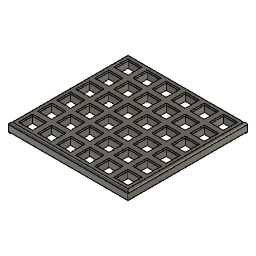
Parametric_Key_Tester (Autodesk Fusion 360 design; units mm, degrees)
part number: Parametric Key Tester
Autodesk Fusion 360 part; units mm, degrees
sketch "Sketch1" plane through (0, 0, 0) normal (0, 0, 1) x (1, 0, 0) in component "Key Tester"
  line L0 (0, 0) -> (119, 0)
  line L1 (119, 0) -> (119, 119)
  line L2 (119, 119) -> (0, 119)
  line L3 (0, 119) -> (0, 0)
  line L4 (5, 5) -> (19, 5)
  line L5 (19, 5) -> (19, 19)
  line L6 (19, 19) -> (5, 19)
  line L7 (5, 19) -> (5, 5)
  line L8 (4, 4) -> (20, 4)
  line L9 (20, 4) -> (20, 20)
  line L10 (20, 20) -> (4, 20)
  line L11 (4, 20) -> (4, 4)
  dimension "d1" = 119
  dimension "d2" = 119
  dimension "d3" = 14
  dimension "d4" = 14
  dimension "d5" = 5
  dimension "d6" = 5
  dimension "d65" = 1
  constraint horizontal L0
  constraint vertical L1
  constraint coincident L0.start L3.end
  constraint horizontal L4
  constraint vertical L5
  constraint horizontal L6
  constraint vertical L7
  constraint horizontal L2
  measures "d1" distance of L0.start L0.end
  measures "d2" distance of L0.start L2.end
  measures "d3" distance of L4.start L4.end
  measures "d4" distance of L4.start L6.end
  measures "d5" distance of L3 L7
  measures "d6" distance of L0 L4
extrude "Extrude6" add sketch "Sketch1" along normal blind 10 contours L0 L1 L2 L3 | L4 L5 L6 L7 | L8 L9 L10 L11 in component "Key Tester"
fillet "Fillet3" radius 2 8 edges at (59.5, 119, 10) (0, 59.5, 10) (59.5, 0, 10) (119, 59.5, 10) (59.5, 119, 0) (119, 59.5, 0) (0, 59.5, 0) (59.5, 0, 0) in component "Key Tester"
extrude "Extrude7" cut sketch "Sketch1" along normal up to surface (10 mm away) contours L4 L5 L6 L7 in component "Key Tester"
extrude "Extrude8" cut sketch "Sketch1" along normal up to surface (8.2 mm away) contours L8 L9 L10 L11 in component "Key Tester"
fillet "Fillet4" radius 1 4 edges at (12, 20, 0) (20, 12, 0) (12, 4, 0) (4, 12, 0) in component "Key Tester"
pattern_linear "R-Pattern1" count 6 spacing 19 along (0, 1, 0) count 6 spacing 19 along (1, 0, 0) of "Extrude7", "Extrude8", "Fillet4" in component "Key Tester"
component "Key Tester" placed x (1, 0, 0) y (0, 1, 0) z (0, 0, 1) at (0, 0, 0)
equation "d1 = SwitchWidth * Columns + SwitchSpacing * Columns + SwitchSpacing"
equation "d2 = SwitchHeight * Rows + SwitchSpacing * Rows + SwitchSpacing"
equation "d3 = SwitchWidth"
equation "d4 = SwitchHeight"
equation "d5 = SwitchSpacing"
equation "d6 = SwitchSpacing"
equation "Rows = 6" comment "Number of rows"
equation "Columns = 6" comment "Number of columns"
equation "SwitchHeight = 14 mm" comment "Switch Height (14 for MX)"
equation "SwitchWidth = 14 mm" comment "Switch Width (14 for MX)"
equation "SwitchSpacing = 5 mm" comment "Spacing between switches (Normally 5)"
equation "d68 = Thickness"
equation "d78 = Rows"
equation "d79 = Columns"
equation "d80 = -( SwitchWidth + SwitchSpacing )"
equation "d81 = -( SwitchWidth + SwitchSpacing )"
equation "Thickness = 10 mm" comment "Thickness of platform"
